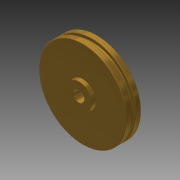
# Autodesk Inventor part: 2in pulley
Saved by Autodesk Inventor 2015 SP1 (Build 190203100, 203)
## iProperties
Created: 2015-01-12
Part Number: 2in pulley
Material: Steel, Alloy
Document SubType Name: Modeling
Designer: Jarod
Density: 7.73 g/cm^3
Appearance: Semi-Polished
Author: Jarod
Autodesk Inventor part; units mm, degrees
ref_plane "YZ Plane" through (0, 0, 0) normal (1, 0, 0) x (0, 1, 0)
ref_plane "XZ Plane" through (0, 0, 0) normal (0, 1, 0) x (-1, 0, 0)
sketch "Sketch1" plane through (0, 0, 0) normal (0, 0, 1) x (1, 0, 0)
  circle A0 centre (0, 0) radius 11.43
  circle A1 centre (0, 0) radius 38.1
  dimension "d0" = 22.86
  dimension "d1" = 76.2
  constraints: 2 centre point, 2 coincident
  measures "d0" diameter of A0
  measures "d1" diameter of A1
extrude "Extrusion1" add sketch "Sketch1" along normal blind 12.7
ref_plane "Work Plane1" through (0, 0, 6.35) normal (0, 0, 1) x (1, 0, 0)
sketch "Sketch3" plane through (0, 0, 6.35) normal (0, 0, 1) x (1, 0, 0)
  circle A0 centre (0, 0) radius 11.1125
  dimension "d9" = 22.225
  constraints: 1 centre point, 1 coincident
  measures "d9" diameter of A0
extrude "Extrusion3" add sketch "Sketch3" along normal mid plane 19.05
sketch "Sketch4" plane through (0, 0, 15.875) normal (0, 0, 1) x (1, 0, 0)
  circle A0 centre (0, 0) radius 4.7625
  dimension "d12" = 9.525
  constraints: 1 centre point, 1 coincident
  measures "d12" diameter of A0
extrude "Extrusion4" cut sketch "Sketch4" against normal blind 25.4
sketch "Sketch5" plane through (0, 0, 6.35) normal (0, 0, 1) x (1, 0, 0)
  circle A0 centre (0, 0) radius 38.1
  circle A1 centre (0, 0) radius 34.925
  circle A2 centre (0, 0) radius 11.43 projected
  circle A3 centre (0, 0) radius 38.1 projected
  dimension "d15" = 3.175
  dimension "d16" = 0
  constraints: 2 centre point, 2 coincident
  measures "d15" radial gap between concentric circles of A0 A1
  measures "d16" radial gap between concentric circles of A0 A3
extrude "Extrusion5" cut sketch "Sketch5" along normal mid plane 3.175 contours A0
fillet "Fillet2" radius 0.7937 6 edges at (-38.1, 0, 0) (-38.1, 0, 4.7625) (-34.925, 0, 4.7625) (-38.1, 0, 12.7) (-38.1, 0, 7.9375) (-34.925, 0, 7.9375)
body "Solid1"
